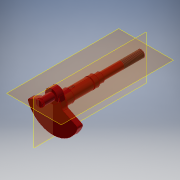
# Autodesk Inventor part: Shaft
Saved by Autodesk Inventor 2018 (Build 220112000, 112)
## iProperties
Created: 2023-03-12
Part Number: Shaft
Material: Generic
Document SubType Name: Modeling
Designer: Habib Mohamed
Density: 1 g/cm^3
Appearance: Red
Author: Habib Mohamed
Autodesk Inventor part; units mm, degrees
ref_plane "YZ Plane" through (0, 0, 0) normal (1, 0, 0) x (0, 1, 0)
ref_plane "XY Plane" through (0, 0, 0) normal (0, 0, 1) x (1, 0, 0)
sketch "Sketch1" plane through (0, 0, 0) normal (1, 0, 0) x (0, 1, 0)
  line L0 (0, 0) -> (11, 0)
  line L1 (11, 0) -> (11, -2.5)
  line L2 (11, -2.5) -> (8.5, -2.5)
  line L3 (8.5, -2.5) -> (8.5, -14.5)
  line L4 (8.5, -14.5) -> (7.5, -14.5)
  line L5 (7.5, -14.5) -> (7.5, -43)
  line L6 (7.5, -43) -> (5, -43)
  line L7 (5, -43) -> (5, -44.25)
  line L8 (5, -44.25) -> (7.5, -44.25)
  line L9 (7.5, -44.25) -> (7.5, -50.5)
  line L10 (7.5, -50.5) -> (6, -50.5)
  line L11 (6, -50.5) -> (6, -58.5)
  line L12 (6, -58.5) -> (5, -58.5)
  line L13 (5, -58.5) -> (5, -115.5)
  line L14 (5, -115.5) -> (0, -115.5)
  line L15 (0, -115.5) -> (0, 0)
  dimension "d0" = 5
  dimension "d1" = 6
  dimension "d2" = 7.5
  dimension "d3" = 5
  dimension "d4" = 8.5
  dimension "d5" = 7.5
  dimension "d6" = 11
  dimension "d7" = 2.5
  dimension "d8" = 12
  dimension "d9" = 1.25
  dimension "d10" = 6.25
  dimension "d12" = 57
  dimension "d13" = 65
  dimension "d14" = 28.5
  constraints: 32 end point, 13 perpendicular, 4 point on line, 1 horizontal
  measures "d0" distance between parallel lines of L15 L13
  measures "d1" distance between parallel lines of L15 L11
  measures "d2" distance between parallel lines of L15 L9
  measures "d3" distance between parallel lines of L15 L7
  measures "d4" distance between parallel lines of L15 L3
  measures "d5" distance between parallel lines of L15 L5
  measures "d6" distance between parallel lines of L15 L1
  measures "d7" distance of L0.end L1.end
  measures "d8" distance of L2.end L3.end
  measures "d9" distance of L6.end L7.end
  measures "d10" distance of L8.end L9.end
  measures "d12" distance of L12.end L13.end
  measures "d13" distance between parallel lines of L10 L14
  measures "d14" distance of L4.end L5.end
revolve "Revolution1" add sketch "Sketch1" angle 360 about axis through (0, 0, -115.5) along (0, 0, 1)
sketch "Sketch2" plane through (0, 0, 0) normal (0, 0, 1) x (1, 0, 0)
  circle A0 centre (0, 10.64) radius 9
  arc A1 (-34.3908, -12.228) -> (34.3908, -12.228) centre (0, 0) ccw
  line L0 (0, 0) -> (118.8939, 0) construction
  line L1 (8.5595, 13.4212) -> (12.3892, 1.6344)
  circle A2 centre (0, 0) radius 5 construction
  line L2 (0, 0) -> (0, 32.7762) construction
  line L3 (14.4714, -0.7398) -> (33.3674, -9.7528)
  line L4 (-8.5595, 13.4212) -> (-12.3892, 1.6344)
  line L5 (-14.4714, -0.7398) -> (-33.3674, -9.7528)
  arc A3 (12.3892, 1.6344) -> (14.4714, -0.7398) centre (16.1935, 2.8705) ccw
  arc A4 (-14.4714, -0.7398) -> (-12.3892, 1.6344) centre (-16.1935, 2.8705) ccw
  arc A5 (34.3908, -12.228) -> (33.3674, -9.7528) centre (32.5064, -11.5579) ccw
  arc A6 (-33.3674, -9.7528) -> (-34.3908, -12.228) centre (-32.5064, -11.5579) ccw
  line L6 (0, 19.64) -> (56.14, 19.64) construction
  line L7 (0, -36.5) -> (89.4441, -36.5) construction
  point P0 (34.9542, -10.5096)
  point P1 (-34.9542, -10.5096)
  point P2 (-12.9203, 0)
  point P3 (12.9203, 0)
  dimension "d16" = 18
  dimension "d17" = 73
  dimension "d18" = 10.64
  dimension "d19" = 18
  dimension "d20" = 25.5
  dimension "d21" = 4
  dimension "d22" = 2
  dimension "d24" = 56.14
  dimension "d25" = 18
  dimension "d26" = 25.5
  constraints: 16 end point, 16 point on circle, 11 tangent, 8 point on line, 6 centre point, 2 equal radius, 2 horizontal, 1 coincident, 1 perpendicular, 1 symmetric about line, 1 vertical
  measures "d16" diameter of A0
  measures "d17" diameter of A1
  measures "d18" distance of A0.centre point (0, 0)
  measures "d19" angle of L1 L2
  measures "d20" angle of L0 L3
  measures "d21" radius of A3
  measures "d22" radius of A5
  measures "d24" distance between parallel lines of L7 L6
  measures "d25" angle of L4 L2
  measures "d26" angle of L5 L0
extrude "Extrusion1" add sketch "Sketch2" along normal blind 7
sketch "Sketch3" plane through (0, 0, 7) normal (0, 0, 1) x (1, 0, 0)
  arc A0 (8.5595, 13.4212) -> (-8.5595, 13.4212) centre (0, 10.64) ccw projected
  circle A1 centre (0, 10.64) radius 9 projected
  point P0 (0, 0)
extrude "Extrusion2" add sketch "Sketch3" along normal blind 1.5
sketch "Sketch4" plane through (0, 10.64, 8.5) normal (0, 0, 1) x (1, 0, 0)
  circle A0 centre (0, 0) radius 5
  point P0 (0, -10.64)
  dimension "d31" = 10
  constraints: 1 centre point
  measures "d31" diameter of A0
extrude "Extrusion3" add sketch "Sketch4" along normal blind 15
sketch "Sketch5" plane through (0, 10.64, 23.5) normal (0, 0, 1) x (1, 0, 0)
  circle A0 centre (0, 0) radius 4.5
  circle A1 centre (0, 0) radius 9 construction
  point P0 (0, -10.64)
  dimension "d35" = 9
  constraints: 1 centre point, 1 coincident
  measures "d35" diameter of A0
extrude "Extrusion4" add sketch "Sketch5" along normal blind 1.1
sketch "Sketch6" plane through (0, 10.64, 24.6) normal (0, 0, 1) x (1, 0, 0)
  circle A0 centre (0, 0) radius 5
  point P0 (0, -10.64)
  dimension "d38" = 10
  constraints: 1 centre point
  measures "d38" diameter of A0
extrude "Extrusion5" add sketch "Sketch6" along normal blind 1.6
chamfer "Chamfer1" distance 0.8 angle 45 1 edges at (-5, 10.64, 26.2) measured on face at (-4.5, 10.64, 26.2)
thread "Thread1" size "M10x1.5" class "6g" standard "ISO Metric profile" length 28
ref_plane "Work Plane1" through (0, 7.5, -28.75) normal (0, 1, 0) x (-1, 0, 0)
sketch "Sketch7" plane through (0, 7.5, -28.75) normal (0, 1, 0) x (-1, 0, 0)
  line L0 (-8.5, 14.25) -> (8.5, 14.25) construction
  line L1 (0, 12.25) -> (0, 7.25) construction
  line L2 (-1.5, 12.25) -> (-1.5, 7.25)
  line L3 (1.5, 7.25) -> (1.5, 12.25)
  arc A0 (1.5, 12.25) -> (-1.5, 12.25) centre (0, 12.25) ccw
  arc A1 (-1.5, 7.25) -> (1.5, 7.25) centre (0, 7.25) ccw
  point P0 (0, 28.75)
  point P1 (0, 9.75)
  dimension "d46" = 1.5
  dimension "d47" = 5
  dimension "d48" = 0.5
  constraints: 8 end point, 4 point on circle, 4 tangent, 2 centre point, 1 midpoint, 1 parallel, 1 vertical
  measures "d46" radius of A1
  measures "d47" distance of L1.start L1.end
  measures "d48" distance edge to line of A0 L0
extrude "Extrusion6" cut sketch "Sketch7" against normal blind 2
body "Solid1"
